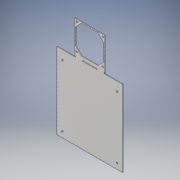
# Autodesk Inventor part: XGEN_hotbed-pcb-org
Saved by Autodesk Inventor 2019 (Build 230136000, 136)
## iProperties
Created: 2019-02-28
Part Number: XGEN_hotbed-pcb-org
Material: Generic
Document SubType Name: Sheet Metal
Designer: Rene
Density: 1 g/cm^3
Sheet Metal Rule: Default_mm
Appearance: Aluminum - Polished
Author: Rene
Autodesk Inventor part; units mm, degrees
ref_plane "YZ Plane" through (0, 0, 0) normal (1, 0, 0) x (0, 1, 0)
ref_plane "XZ Plane" through (0, 0, 0) normal (0, 1, 0) x (-1, 0, 0)
ref_plane "XY Plane" through (0, 0, 0) normal (0, 0, 1) x (1, 0, 0)
sketch "Sketch1" plane through (0, 0, 0) normal (0, 0, 1) x (1, 0, 0)
  line L0 (-90, -105) -> (90, -105)
  line L1 (90, -105) -> (90, 105)
  line L2 (-90, 105) -> (-90, -105)
  line L3 (42, 105) -> (42, 197)
  line L4 (42, 197) -> (-42, 197)
  line L5 (-42, 197) -> (-42, 105)
  line L6 (90, 105) -> (42, 105)
  line L7 (-42, 105) -> (-90, 105)
  point P0 (0, 0)
  dimension "d0" = 180
  dimension "d1" = 210
  dimension "d2" = 105
  dimension "d3" = 90
  dimension "d22" = 92
  dimension "d24" = 42
  dimension "d26" = 84
  dimension "d28" = 92
  dimension "d29" = 210
  dimension "d30" = 48
  dimension "d31" = 48
  constraints: 16 end point, 4 parallel, 1 horizontal, 1 perpendicular
  measures "d0" distance of L0.start L0.end
  measures "d1" distance of L2.start L0.start
  measures "d2" vertical distance of point (0, 0) L0.start
  measures "d3" horizontal distance of point (0, 0) L0.start
  measures "d22" distance of L4.end L5.end
  measures "d24" horizontal distance of point (0, 0) L4.end
  measures "d26" distance of L3.end L4.end
  measures "d28" distance of L3.start L3.end
  measures "d29" distance of L0.end L1.end
  measures "d30" distance of L5.end L2.start
  measures "d31" distance of L1.end L3.start
extrude "Extrusion1" add sketch "Sketch1" along normal blind 2
sketch "Sketch2" plane through (0, 0, 2) normal (0, 0, 1) x (1, 0, 0)
  line L0 (-90, -105) -> (90, -105) projected
  line L1 (-42, 105) -> (-90, 105) projected
  point P0 (0, 0)
  point P1 (-75, 80)
  point P2 (75, 80)
  point P3 (-75, -90)
  point P4 (75, -90)
  dimension "d6" = 170
  dimension "d8" = 150
  dimension "d9" = 75
  dimension "d10" = 150
  dimension "d11" = 15
  dimension "d12" = 15
  dimension "d13" = 170
  dimension "d14" = 75
  dimension "d27" = 25
  measures "d6" distance of point (-75, 80) point (-75, -90)
  measures "d8" distance of point (75, -90) point (-75, -90)
  measures "d9" horizontal distance of point (0, 0) point (-75, -90)
  measures "d10" distance of point (75, 80) point (-75, 80)
  measures "d11" distance from line of point (-75, -90) L0
  measures "d12" distance from line of point (75, -90) L0
  measures "d13" distance of point (75, 80) point (75, -90)
  measures "d14" horizontal distance of point (0, 0) point (-75, 80)
  measures "d27" distance from line of L1 point (-75, 80)
hole "Hole1" at (-75, 80, 2) at (75, 80, 2) at (-75, -90, 2) at (75, -90, 2) direction (0, 0, -1) diameter 4.2 end through all
sketch "Sketch3" plane through (0, 0, 2) normal (0, 0, 1) x (1, 0, 0)
  line L0 (-90, 105) -> (-90, -105) projected
  line L1 (90, 105) -> (42, 105) projected
  line L2 (-39, 116) -> (39, 116)
  line L3 (39, 116) -> (39, 194)
  line L4 (39, 194) -> (-39, 194)
  line L5 (-39, 194) -> (-39, 116)
  point P0 (0, 0)
  dimension "d46" = 78
  dimension "d47" = 39
  dimension "d48" = 78
  dimension "d49" = 11
  constraints: 8 end point, 2 parallel, 1 horizontal, 1 perpendicular
  measures "d46" distance of L2.end L2.start
  measures "d47" horizontal distance of point (0, 0) L2.start
  measures "d48" distance of L4.end L2.start
  measures "d49" vertical distance of L2.start L0.start
extrude "Extrusion2" cut sketch "Sketch3" against normal blind 10
chamfer "Chamfer1" distance 16.5 angle 45 4 edges at (-39, 116, 1) (39, 116, 1) (-39, 194, 1) (39, 194, 1)
sketch "Sketch4" plane through (0, 0, 2) normal (0, 0, 1) x (1, 0, 0)
  line L0 (-35.75, 190.9) -> (35.75, 190.9) construction
  line L1 (35.75, 190.9) -> (35.75, 119.4) construction
  line L2 (35.75, 119.4) -> (-35.75, 119.4) construction
  line L3 (-35.75, 119.4) -> (-35.75, 190.9) construction
  line L4 (90, 105) -> (42, 105) construction
  point P0 (0, 0)
  dimension "d53" = 71.5
  dimension "d54" = 35.75
  dimension "d55" = 71.5
  dimension "d56" = 14.4
  constraints: 8 end point, 4 coincident, 2 parallel, 1 horizontal, 1 perpendicular
  measures "d53" distance of L1.end L2.end
  measures "d54" horizontal distance of point (0, 0) L2.end
  measures "d55" distance of L2.end L0.start
  measures "d56" distance from line of L4 L1.end
hole "Hole2" at (-35.75, 190.9, 2) at (35.75, 190.9, 2) at (-35.75, 119.4, 2) at (35.75, 119.4, 2) direction (0, 0, -1) diameter 4.2 end through all
sketch "Sketch5" plane through (0, 0, 2) normal (0, 0, 1) x (1, 0, 0)
  line L0 (-42, 197) -> (-42, 105) projected
  line L1 (-42, 105) -> (-39, 105)
  line L2 (-39, 105) -> (-39, 107)
  line L3 (-39, 107) -> (-42, 107)
  line L4 (-42, 107) -> (-42, 105)
  line L5 (90, 105) -> (42, 105) projected
  line L6 (42, 105) -> (39, 105)
  line L7 (39, 105) -> (39, 107)
  line L8 (39, 107) -> (42, 107)
  line L9 (42, 107) -> (42, 105)
  line L10 (-20, 105) -> (20, 105)
  line L11 (20, 105) -> (20, 107)
  line L12 (20, 107) -> (-20, 107)
  line L13 (-20, 107) -> (-20, 105)
  point P0 (0, 0)
  dimension "d64" = 2
  dimension "d65" = 2
  dimension "d66" = 2
  dimension "d67" = 3
  dimension "d68" = 3
  dimension "d69" = 40
  dimension "d70" = 20
  constraints: 24 end point, 6 parallel, 3 horizontal, 3 perpendicular, 3 point on line
  measures "d64" distance between parallel lines of L3 L1
  measures "d65" distance between parallel lines of L12 L10
  measures "d66" distance between parallel lines of L8 L6
  measures "d67" distance of L0.end L1.end
  measures "d68" distance of L5.end L6.end
  measures "d69" distance of L10.end L10.start
  measures "d70" horizontal distance of point (0, 0) L10.start
extrude "Extrusion3" cut sketch "Sketch5" against normal blind 10
fillet "Fillet1" radius 1 8 edges at (-39, 105, 1) (-39, 107, 1) (-20, 107, 1) (-20, 105, 1) (20, 105, 1) (20, 107, 1) (39, 107, 1) (39, 105, 1)
equation "\"d2\" = 0.5 * d1"
equation "\"d3\" = 0.5 * d0"
equation "\"d24\" = 0.5 * d26"
equation "\"d28\" = d22"
equation "\"d9\" = 0.5 * d8"
equation "\"d10\" = d8"
equation "\"d12\" = d11"
equation "\"d13\" = d6"
equation "\"d14\" = d9"
equation "\"d20\" = Thickness"
equation "\"d47\" = 0.5 * d46"
equation "\"d48\" = d46"
equation "\"d54\" = 0.5 * d53"
equation "\"d55\" = d53"
equation "\"d62\" = Thickness"
equation "\"d70\" = 0.5 * d69"
equation "\"BendRadius\" = Thickness"
equation "\"BendReliefWidth\" = Thickness"
equation "\"BendReliefDepth\" = 0.5 * Thickness"
equation "\"CornerReliefSize\" = 4 * Thickness"
equation "\"MinimumRemnant\" = 2 * Thickness"
equation "\"TransitionRadius\" = BendRadius"
equation "\"JacobiRadiusSize\" = BendRadius"
equation "\"GapSize\" = Thickness"
equation "\"Thickness\" = 0.5"
body "Solid1"
